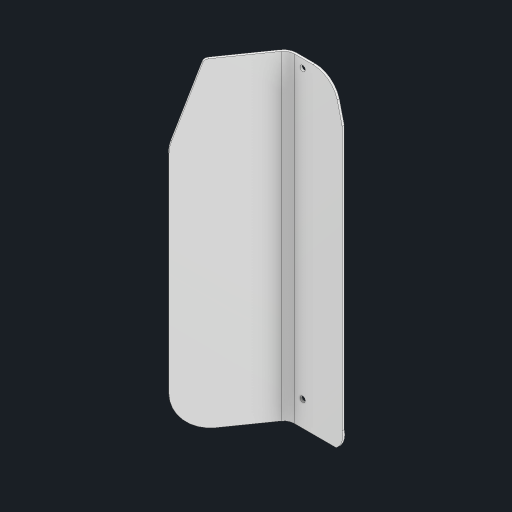
# Autodesk Inventor part: wedge
Saved by Autodesk Inventor 2024 (Build 280153000, 153)
## iProperties
Created: 2023-08-19
Part Number: wedge
Material: Acetal Resin, White
Document SubType Name: Modeling
Designer: Averey
Density: 1.425 g/cm^3
Appearance: Smooth - White
Author: Averey
Autodesk Inventor part; units mm, degrees
note: some values were not read from the file. Chosen so that the rebuilt part matches the saved one: bend side of "Bend Part1".
ref_plane "YZ Plane" through (0, 0, 0) normal (1, 0, 0) x (0, 1, 0)
ref_plane "XZ Plane" through (0, 0, 0) normal (0, 1, 0) x (-1, 0, 0)
ref_plane "XY Plane" through (0, 0, 0) normal (0, 0, 1) x (1, 0, 0)
sketch "Sketch1" plane through (0, 0, 0) normal (0, 0, 1) x (1, 0, 0)
  circle A0 centre (-3.1769, 113.7672) radius 2.0955
  circle A1 centre (-3.1769, -102.1328) radius 2.0955
  line L0 (-9.5269, 120.1172) -> (4.5684, 120.1172)
  line L1 (-9.5269, -121.1828) -> (-9.5269, 120.1172)
  line L2 (-9.5269, 120.1172) -> (-58.0591, 120.1172)
  line L3 (-79.3769, 60.3213) -> (-79.3769, -95.7828)
  line L4 (-9.5269, -121.1828) -> (-9.5269, 120.1172)
  line L5 (-61.0624, 117.9719) -> (-78.0039, 68.5592)
  arc A2 (-78.0039, 68.5592) -> (-79.3769, 60.3213) centre (-53.9769, 60.3213) ccw
  arc A3 (-79.3769, -95.7828) -> (-53.9769, -121.1828) centre (-53.9769, -95.7828) ccw
  arc A4 (-58.0591, 120.1172) -> (-61.0624, 117.9719) centre (-58.0591, 116.9422) ccw
  arc A5 (22.9235, 106.1658) -> (4.5684, 120.1172) centre (4.5684, 101.0672) ccw
  arc A6 (22.2231, -121.1828) -> (26.6067, -107.95) centre (14.337, -111.228) ccw
  line L6 (-41.2769, -121.1828) -> (22.2231, -121.1828)
  line L7 (26.6067, -107.95) -> (26.6067, 90.8579)
  line L8 (22.9235, 106.1658) -> (26.6067, 90.8579)
  line L9 (-53.9769, -121.1828) -> (-41.2769, -121.1828)
  point P0 (0, 0)
  point P1 (-79.3769, -121.1828)
  dimension "d0" = 4.191
  dimension "d1" = 4.191
  dimension "d2" = 69.85
  dimension "d3" = 25.4
  dimension "d4" = 3.175
  dimension "d5" = 19.05
  dimension "d16" = 12.7
  dimension "d18" = 63.5
  constraints: 20 end point, 10 point on circle, 7 centre point, 7 tangent, 4 horizontal, 3 vertical, 2 point on line, 1 collinear, 1 equal radius, 1 parallel, 1 perpendicular, 1 other
  measures "d0" diameter of A0
  measures "d1" diameter of A1
  measures "d2" distance of L1.start point (-79.377, -121.183)
  measures "d3" radius of A2
  measures "d4" radius of A4
  measures "d5" radius of A5
  measures "d16" radius of A6
  measures "d18" distance of L6.start L6.end
extrude "Extrusion1" add sketch "Sketch1" along normal blind 1.5875
bend part "Bend Part1" radius 9.525 angle 55 line through (-9.5269, -121.1828, 0) along (0, 1, 0) centre toward (0, 0, 1) moving side (-1, 0, 0) both sides no
body "Solid1"
